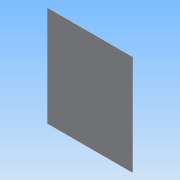
# Autodesk Inventor part: TopPanel
Saved by Autodesk Inventor 2014 (Build 180170000, 170)
## iProperties
Created: 2014-01-06
Part Number: TopPanel
Material: ABS Plastic
Document SubType Name: Modeling
Designer: davidgitz
Density: 1 g/cm^3
Appearance: Smooth - White
Author: davidgitz
Autodesk Inventor part; units mm, degrees
ref_plane "YZ Plane" through (0, 0, 0) normal (1, 0, 0) x (0, 1, 0)
ref_plane "XZ Plane" through (0, 0, 0) normal (0, 1, 0) x (-1, 0, 0)
ref_plane "XY Plane" through (0, 0, 0) normal (0, 0, 1) x (1, 0, 0)
sketch "Sketch1" plane through (0, 0, 0) normal (0, 0, 1) x (1, 0, 0)
  line L0 (-123.3338, -12.7) -> (-123.3338, 6.35) projected
  line L1 (123.3338, -12.7) -> (-123.3338, -12.7) projected
  line L2 (123.3338, -12.7) -> (123.3338, 6.35) projected
  line L3 (123.3338, -266.7) -> (123.3338, -285.75) projected
  line L4 (-123.3338, -266.7) -> (123.3338, -266.7) projected
  line L5 (-123.3338, -266.7) -> (-123.3338, -285.75) projected
  line L6 (123.3338, 6.35) -> (-123.3338, 6.35)
  line L7 (-123.3338, 6.35) -> (-123.3338, -285.75)
  line L8 (-123.3338, -285.75) -> (123.3338, -285.75)
  line L9 (123.3338, -285.75) -> (123.3338, 6.35)
  line L10 (123.3338, 6.35) -> (-123.3338, 6.35) projected
  line L11 (-123.3338, -285.75) -> (123.3338, -285.75) projected
  point P0 (0, 0)
  constraints: 8 end point, 2 parallel, 1 horizontal, 1 perpendicular
extrude "Extrusion1" add sketch "Sketch1" along normal blind 1.5875
body "Solid1"
